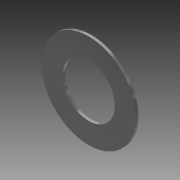
# Autodesk Inventor part: Thrust Bearing Washer - .7500 Bore
Saved by Autodesk Inventor 2014 SP1 (Build 180222100, 222)
## iProperties
Created: 2013-06-04
Part Number: Thrust Bearing Washer - .7500 Bore
Material: Stainless Steel
Document SubType Name: Modeling
Designer: mvarma
Density: 8.08 g/cm^3
Mass: 2.84355 g
Surface Area: 9.9758 cm^2
Volume: 0.351924 cm^3
Appearance: Semi-Polished
Author: mvarma
Autodesk Inventor part; units mm, degrees
ref_plane "YZ Plane" through (0, 0, 0) normal (1, 0, 0) x (0, 1, 0)
ref_plane "XZ Plane" through (0, 0, 0) normal (0, 1, 0) x (-1, 0, 0)
ref_plane "XY Plane" through (0, 0, 0) normal (0, 0, 1) x (1, 0, 0)
sketch "Sketch1" plane through (0, 0, 0) normal (0, 0, 1) x (1, 0, 0)
  circle A0 centre (0, 0) radius 7.9375
  circle A1 centre (0, 0) radius 14.2875
  dimension "d0" = 15.875
  dimension "d1" = 28.575
  constraints: 2 centre point, 2 coincident
  measures "d0" diameter of A0
  measures "d1" diameter of A1
extrude "Extrusion1" add sketch "Sketch1" along normal blind 0.7937
body "Solid1"
